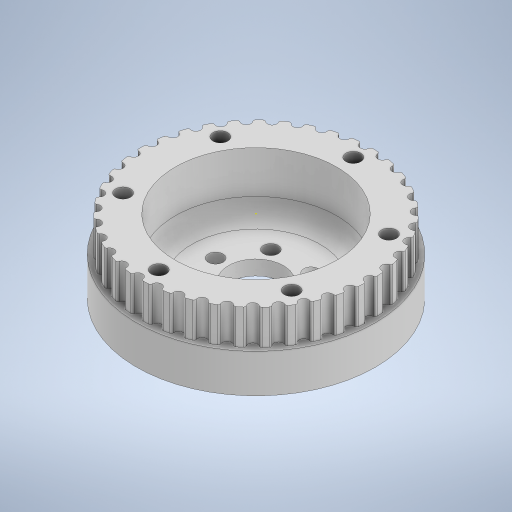
# Autodesk Inventor part: OnPatronFlanech
Saved by Autodesk Inventor 2024 (Build 280153000, 153)
## iProperties
Created: 2023-08-26
Part Number: OnPatronFlanech
Material: Generic
Document SubType Name: Modeling
Designer: KirikDK
Density: 1 g/cm^3
Appearance: Default
Author: KirikDK
Autodesk Inventor part; units mm, degrees
ref_plane "YZ Plane" through (0, 0, 0) normal (1, 0, 0) x (0, 1, 0)
ref_plane "XZ Plane" through (0, 0, 0) normal (0, 1, 0) x (-1, 0, 0)
ref_plane "XY Plane" through (0, 0, 0) normal (0, 0, 1) x (1, 0, 0)
sketch "Sketch1" plane through (0, 0, 0) normal (0, 1, 0) x (-1, 0, 0)
  circle A0 centre (0, 0) radius 62.5
  circle A1 centre (0, 0) radius 53
  circle A2 centre (0, -53) radius 4.05
  circle A3 centre (0, 0) radius 44
  circle A4 centre (45.8993, -26.5) radius 4.05
  circle A5 centre (45.8993, 26.5) radius 4.05
  circle A6 centre (0, 53) radius 4.05
  circle A7 centre (-45.8993, 26.5) radius 4.05
  circle A8 centre (-45.8993, -26.5) radius 4.05
  dimension "d1" = 106
  dimension "d0" = 125
  dimension "d4" = 360
  dimension "d18" = 8.1
  constraints: 8 centre point, 3 coincident, 1 vertical alignment, 15 other
  measures "d0" diameter of A0
  measures "d18" diameter of A2
extrude "Extrusion1" add sketch "Sketch1" along normal blind 8 contours A0 | A1 A4 A2 A8 A7 A6 A5
sketch "Sketch2" plane through (0, 8, 0) normal (0, 1, 0) x (1, 0, 0)
  circle A0 centre (0, 0) radius 44 projected
  circle A1 centre (0, 0) radius 15
  circle A2 centre (-22, 0) radius 4.05
  circle A3 centre (-11, -19.0526) radius 4.05
  circle A4 centre (11, -19.0526) radius 4.05
  circle A5 centre (22, 0) radius 4.05
  circle A6 centre (11, 19.0526) radius 4.05
  circle A7 centre (-11, 19.0526) radius 4.05
  dimension "d8" = 30
  dimension "d11" = 22
  dimension "d12" = 8.1
  dimension "d15" = 360
  constraints: 7 centre point, 1 coincident, 13 other
  measures "d8" diameter of A1
  measures "d11" distance of point (0, 0) A2.centre
  measures "d12" diameter of A2
extrude "Extrusion2" add sketch "Sketch2" against normal blind 8
sketch "Sketch3" plane through (0, 8, 0) normal (0, 1, 0) x (1, 0, 0)
  circle A0 centre (0, 0) radius 30
  circle A1 centre (0, 0) radius 15 projected
  circle A2 centre (-22, 0) radius 4.05 projected
  circle A3 centre (-11, -19.0526) radius 4.05 projected
  circle A4 centre (11, -19.0526) radius 4.05 projected
  circle A5 centre (22, 0) radius 4.05 projected
  circle A6 centre (11, 19.0526) radius 4.05 projected
  circle A7 centre (-11, 19.0526) radius 4.05 projected
  circle A8 centre (0, 0) radius 62.5 projected
  circle A9 centre (0, 53) radius 4.05 projected
  circle A10 centre (-45.8993, 26.5) radius 4.05 projected
  circle A11 centre (-45.8993, -26.5) radius 4.05 projected
  circle A12 centre (0, -53) radius 4.05 projected
  circle A13 centre (45.8993, -26.5) radius 4.05 projected
  circle A14 centre (45.8993, 26.5) radius 4.05 projected
  dimension "d17" = 60
  constraints: 1 centre point, 1 coincident
  measures "d17" diameter of A0
extrude "Extrusion3" add sketch "Sketch3" along normal blind 20 contours A0
sketch "Sketch4" plane through (0, 8, 0) normal (0, 1, 0) x (1, 0, 0)
  circle A0 centre (0, 0) radius 46.75
  circle A1 centre (0, 0) radius 44 projected
  circle A2 centre (0, 0) radius 30 projected
  circle A3 centre (0, 0) radius 62.5 projected
  circle A4 centre (0, 53) radius 4.05 projected
  circle A5 centre (-45.8993, 26.5) radius 4.05 projected
  circle A6 centre (-45.8993, -26.5) radius 4.05 projected
  circle A7 centre (0, -53) radius 4.05 projected
  circle A8 centre (45.8993, -26.5) radius 4.05 projected
  circle A9 centre (45.8993, 26.5) radius 4.05 projected
  dimension "d24" = 93.5
  constraints: 1 centre point, 1 coincident
  measures "d24" diameter of A0
extrude "Extrusion4" add sketch "Sketch4" along normal blind 7 contours A0 | A1
sketch "Sketch5" plane through (0, 28, 0) normal (0, 1, 0) x (1, 0, 0)
  circle A0 centre (0, 0) radius 30 projected
  circle A1 centre (-11, 19.0526) radius 4.05 projected
  circle A2 centre (11, 19.0526) radius 4.05 projected
  circle A3 centre (22, 0) radius 4.05 projected
  circle A4 centre (11, -19.0526) radius 4.05 projected
  circle A5 centre (-11, -19.0526) radius 4.05 projected
  circle A6 centre (-22, 0) radius 4.05 projected
  circle A7 centre (0, 0) radius 15 projected
extrude "Extrusion5" add sketch "Sketch5" along normal blind 2
sketch "Sketch6" plane through (0, 30, 0) normal (0, 1, 0) x (1, 0, 0)
  circle A0 centre (0, 0) radius 73.0274
  constraints: 1 centre point, 1 coincident
extrude "Extrusion6" cut sketch "Sketch6" against normal blind 22
sketch "Sketch7" plane through (0, 8, 0) normal (0, 1, 0) x (1, 0, 0)
  circle A0 centre (-11, 19.0526) radius 4.05 projected
  circle A1 centre (11, 19.0526) radius 4.05 projected
  circle A2 centre (22, 0) radius 4.05 projected
  circle A3 centre (11, -19.0526) radius 4.05 projected
  circle A4 centre (-11, -19.0526) radius 4.05 projected
  circle A5 centre (-22, 0) radius 4.05 projected
  circle A6 centre (0, 0) radius 15 projected
  circle A7 centre (0, 0) radius 62.5 projected
  circle A8 centre (0, 53) radius 4.05 projected
  circle A9 centre (-45.8993, 26.5) radius 4.05 projected
  circle A10 centre (-45.8993, -26.5) radius 4.05 projected
  circle A11 centre (0, -53) radius 4.05 projected
  circle A12 centre (45.8993, -26.5) radius 4.05 projected
  circle A13 centre (45.8993, 26.5) radius 4.05 projected
extrude "Extrusion7" add sketch "Sketch7" along normal blind 32
sketch "Sketch8" plane through (0, 40, 0) normal (0, 1, 0) x (1, 0, 0)
  circle A0 centre (0, 0) radius 44
  constraints: 1 centre point, 1 coincident
extrude "Extrusion8" cut sketch "Sketch8" against normal blind 32
sketch "Sketch9" plane through (0, 40, 0) normal (0, 1, 0) x (1, 0, 0)
  circle A0 centre (61.9, 0) radius 2.55
  point P0 (0, 0)
  dimension "d39" = 5.1
  dimension "d44" = 61.9
  constraints: 1 centre point
  measures "d39" diameter of A0
  measures "d44" distance of point (0, 0) A0.centre
extrude "Extrusion9" cut sketch "Sketch9" against normal blind 19
pattern_circular "Circular Pattern1" count 39 over 360 about axis through (0, 8, 0) along (0, -1, 0) of "Extrusion9"
fillet "Fillet1" radius 9 1 edges at (-44, 8, 0)
sketch "Sketch10" plane through (0, 0, 0) normal (0, -1, 0) x (1, 0, 0)
  arc A0 (5.0558, 62.2952) -> (-0.0267, 62.5) centre (0, 0) ccw projected
  circle A1 centre (0, 0) radius 62.5
  circle A2 centre (0, 0) radius 65
  point P0 (5.0558, 62.2952)
  dimension "d40" = 125
  dimension "d41" = 130
  constraints: 2 coincident, 1 centre point, 3 other
  measures "d41" diameter of A2
extrude "Extrusion10" add sketch "Sketch10" against normal blind 21
fillet "Fillet2" radius 1 78 edges at (-0.0267, 30.5, 62.5) (5.0558, 30.5, 62.2952) (9.9993, 30.5, 61.6949) (14.9832, 30.5, 60.6775) (19.7664, 30.5, 59.292) (24.5225, 30.5, 57.4882) (29.0215, 30.5, 55.3534) (33.4267, 30.5, 52.8101) (37.525, 30.5, 49.9812) (41.4652, 30.5, 46.7642) (45.0566, 30.5, 43.3146) (48.4297, 30.5, 39.5071) (51.4213, 30.5, 35.5261) (54.14, 30.5, 31.2268) (56.4542, 30.5, 26.8174) (58.448, 30.5, 22.1378) (-56.4771, 30.5, 26.7691) (-54.1132, 30.5, 31.2732) (-48.3959, 30.5, 39.5486) (-51.4517, 30.5, 35.482) (-41.4251, 30.5, 46.7997) (-37.5678, 30.5, 49.9491) (-33.3815, 30.5, 52.8387) (-29.0689, 30.5, 55.3286) (-24.4733, 30.5, 57.5092) (-19.8171, 30.5, 59.2751) (-14.9313, 30.5, 60.6903) (-61.2316, 30.5, -12.5278) (-62.0475, 30.5, -7.507) (-62.0475, 30.5, 7.507) (-61.2316, 30.5, 12.5278) (-58.429, 30.5, -22.1878) (-60.0398, 30.5, -17.3629) (-60.0398, 30.5, 17.3629) (-58.429, 30.5, 22.1878) (-45.0937, 30.5, 43.276) (-10.0521, 30.5, 61.6863) (-5.0025, 30.5, 62.2995) (62.4504, 30.5, 2.4899) (61.2423, 30.5, 12.4754) (62.4504, 30.5, -2.4899) (62.0411, 30.5, -7.5601) (41.4652, 30.5, -46.7642) (56.4542, 30.5, -26.8174) (60.0249, 30.5, -17.4143) (45.0566, 30.5, -43.3146) (54.14, 30.5, -31.2268) (24.5225, 30.5, -57.4882) (-62.4482, 30.5, -2.5433) (-62.4482, 30.5, 2.5433) (60.0249, 30.5, 17.4143) (29.0215, 30.5, -55.3534) (5.0558, 30.5, -62.2952) (-0.0267, 30.5, -62.5) (14.9832, 30.5, -60.6775) (9.9993, 30.5, -61.6949) (33.4267, 30.5, -52.8101) (19.7664, 30.5, -59.292) (-37.5678, 30.5, -49.9491) (-5.0025, 30.5, -62.2995) (-10.0521, 30.5, -61.6863) (-14.9313, 30.5, -60.6903) (-19.8171, 30.5, -59.2751) (-24.4733, 30.5, -57.5092) (-29.0689, 30.5, -55.3286) (-56.4771, 30.5, -26.7691) (-54.1132, 30.5, -31.2732) (-41.4251, 30.5, -46.7997) (-45.0937, 30.5, -43.276) (-51.4517, 30.5, -35.482) (-33.3815, 30.5, -52.8387) (-48.3959, 30.5, -39.5486) (61.2423, 30.5, -12.4754) (62.0411, 30.5, 7.5601) (48.4297, 30.5, -39.5071) (51.4213, 30.5, -35.5261) (37.525, 30.5, -49.9812) (58.448, 30.5, -22.1378)
sketch "Sketch11" plane through (0, 40, 0) normal (0, 1, 0) x (1, 0, 0)
  point P0 (0, 0)
body "Solid1"
